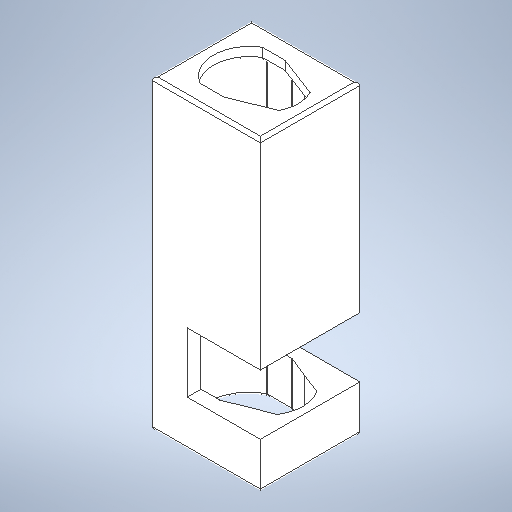
# Autodesk Inventor part: PipetteSleeve
Saved by Autodesk Inventor 2025.1 (Build 291241000, 241)
## iProperties
Created: 2024-10-27
Part Number: PipetteSleeve
Material: Generic
Document SubType Name: Modeling
Designer: 13156
Density: 1 g/cm^3
Appearance: Default
Author: 13156
## iProperties of the stored document PipetteSleeve_3DPrint.ipt
Created: 2024-10-27
Part Number: PipetteSleeve_3DPrint
Material: Generic
Document SubType Name: Modeling
Designer: jerem
Density: 1 g/cm^3
Appearance: Default
Author: jerem
Autodesk Inventor part; units mm, degrees
ref_plane "YZ Plane" through (0, 0, 0) normal (1, 0, 0) x (0, 1, 0)
ref_plane "XZ Plane" through (0, 0, 0) normal (0, 1, 0) x (-1, 0, 0)
ref_plane "XY Plane" through (0, 0, 0) normal (0, 0, 1) x (1, 0, 0)
sketch "Sketch1" plane through (0, 0, 0) normal (0, 1, 0) x (-1, 0, 0)
  arc A0 (11.078, -10.268) -> (11.078, 14.332) centre (5.1039, 2.032) ccw
  line L0 (11.078, -21.6994) -> (11.078, 25.4698)
  line L1 (11.078, 14.332) -> (2.478, 14.332)
  line L2 (11.078, -10.268) -> (2.478, -10.268)
  line L3 (2.478, 14.332) -> (-4.322, 11.532)
  line L4 (2.478, -10.268) -> (-4.322, -7.468)
  line L5 (-4.322, 11.532) -> (-11.422, 8.832)
  line L6 (-4.322, -7.468) -> (-11.422, -4.768)
  arc A1 (-11.422, 8.832) -> (-11.422, -4.768) centre (-0.862, 2.032) ccw
  line L7 (21.1018, 19.039) -> (-15.8982, 19.039)
  line L8 (-15.8982, 19.039) -> (-15.8982, -14.961)
  line L9 (-15.8982, -14.961) -> (21.1018, -14.961)
  line L10 (21.1018, -14.961) -> (21.1018, 19.039)
  point P0 (0, 0)
  point P1 (11.078, 2.032)
  point P2 (18.778, 2.032)
  point P3 (-13.422, 2.032)
  dimension "d0" = 0
  dimension "d1" = 0
  dimension "d2" = 7.7
  dimension "d3" = 8.6
  dimension "d4" = 8.6
  dimension "d5" = 2.8
  dimension "d6" = 2.8
  dimension "d7" = 6.8
  dimension "d8" = 6.8
  dimension "d9" = 24.6
  dimension "d10" = 7.1
  dimension "d11" = 7.1
  dimension "d12" = 2.7
  dimension "d13" = 2.7
  dimension "d14" = 2
  dimension "d56" = 34
  dimension "d57" = 37
  constraints: 22 end point, 6 point on circle, 3 horizontal, 2 centre point, 2 parallel, 1 perpendicular
  measures "d0" vertical distance of point (18.778, 2.032) point (11.078, 2.032)
  measures "d1" distance from line of L0 L1.start
  measures "d2" distance from line of L0 point (18.778, 2.032)
  measures "d3" distance of L1.start L1.end
  measures "d4" distance of L2.start L2.end
  measures "d5" vertical distance of L3.end L1.end
  measures "d6" vertical distance of L4.end L2.end
  measures "d7" horizontal distance of L4.end L2.end
  measures "d8" horizontal distance of L3.end L1.end
  measures "d9" distance of L2.start L1.start
  measures "d10" horizontal distance of L5.end L3.end
  measures "d11" horizontal distance of L6.end L4.end
  measures "d12" vertical distance of L4.end L6.end
  measures "d13" vertical distance of L3.end L5.end
  measures "d14" horizontal distance of L6.end point (-13.422, 2.032)
  measures "d56" distance of L7.end L8.end
  measures "d57" distance of L8.end L9.end
extrude "Extrusion1" add sketch "Sketch1" along normal blind 104.4 contours A0 L0 L7 L10 L9 | L0 L9 L8 L7 L1 L3 L5 A1 L6 L4 L2
sketch "Sketch3" plane through (0, 104.4, 0) normal (0, 1, 0) x (1, 0, 0)
  line L0 (-11.078, -12.682) -> (-2.8044, -12.682)
  line L1 (-2.8044, -12.682) -> (3.6938, -10.0063)
  line L2 (4.322, -11.532) -> (-2.478, -14.332) projected
  line L3 (3.6938, -10.0063) -> (10.43, -7.2326)
  line L4 (10.43, 3.38) -> (-3.3441, 8.618)
  line L5 (-3.3441, 8.618) -> (-11.078, 8.618)
  arc A0 (-11.078, 8.618) -> (-11.078, -12.682) centre (-4.7292, -2.032) ccw
  arc A1 (10.43, -7.2326) -> (10.43, 3.38) centre (0.611, -1.9263) ccw
  line L6 (-2.478, -14.332) -> (-11.078, -14.332) projected
  line L7 (-11.078, 10.268) -> (-2.478, 10.268) projected
  line L8 (4.322, 7.468) -> (11.422, 4.768) projected
  arc A2 (11.422, -8.832) -> (11.422, 4.768) centre (0.862, -2.032) ccw projected
  arc A3 (-11.078, 10.268) -> (-11.078, -14.332) centre (-5.1039, -2.032) ccw projected
  line L9 (-19.5547, -18.0128) -> (14.794, -18.0128)
  line L10 (14.794, -18.0128) -> (14.794, 13.635)
  line L11 (14.794, 13.635) -> (-19.5547, 13.635)
  line L12 (-19.5547, 13.635) -> (-19.5547, -18.0128)
  point P0 (0, 0)
  point P1 (13.422, -2.032)
  point P2 (11.772, -1.9263)
  point P3 (-17.128, -2.032)
  point P4 (-18.778, -2.032)
  dimension "d31" = 1.65
  dimension "d32" = 1.65
  dimension "d33" = 1.65
  dimension "d34" = 180
  dimension "d35" = 1.65
  dimension "d36" = 1.65
  dimension "d37" = 1.65
  dimension "d38" = 0
  constraints: 18 end point, 8 point on circle, 3 horizontal, 3 parallel, 2 centre point, 1 perpendicular, 1 point on line
  measures "d31" distance between parallel lines of L6 L0
  measures "d32" distance between parallel lines of L7 L5
  measures "d33" distance between parallel lines of L1 L2
  measures "d34" angle of L8 L4
  measures "d35" distance from line of L8 L4.start
  measures "d36" horizontal distance of point (13.422, -2.032) point (11.772, -1.926)
  measures "d37" distance of point (-17.128, -2.032) point (-18.778, -2.032)
  measures "d38" horizontal distance of L4.start L3.end
extrude "Extrusion2" add sketch "Sketch3" against normal blind 4
fillet "Fillet2" radius 1 8 edges at (-2.6018, 0, 19.039) (-21.1018, 0, 2.039) (15.8982, 0, 2.039) (-2.6018, 0, -14.961) (-2.6018, 104.4, -14.961) (-21.1018, 104.4, 2.039) (-2.6018, 104.4, 19.039) (15.8982, 104.4, 2.039)
fillet "Fillet3" radius 1 22 edges at (-18.778, 0, 2.032) (-6.778, 0, -10.268) (-6.778, 0, 14.332) (0.922, 0, 12.932) (7.872, 0, 10.182) (13.422, 0, 2.032) (7.872, 0, -6.118) (0.922, 0, -8.868) (-17.128, 100.4, 2.032) (-7.211, 100.4, -8.618) (3.5429, 100.4, -5.999) (11.772, 100.4, 1.9263) (-6.9412, 100.4, 12.682) (3.8128, 100.4, 9.9573) (-11.078, 50.2, 14.332) (-2.478, 50.2, 14.332) (4.322, 50.2, 11.532) (11.422, 50.2, 8.832) (11.422, 50.2, -4.768) (4.322, 50.2, -7.468) (-2.478, 50.2, -10.268) (-11.078, 50.2, -10.268)
sketch "Sketch5" plane through (15.8982, 1, 19.039) normal (1, 0, 0) x (0, 0, -1)
  line L0 (39, 35.2) -> (-4, 35.2)
  line L1 (-4, 35.2) -> (-4, 14.7)
  line L2 (-4, 14.7) -> (39, 14.7)
  line L3 (39, 14.7) -> (39, 35.2)
  line L4 (34, 0) -> (34, 102.4) projected
  line L5 (33, 103.4) -> (1, 103.4) projected
  point P0 (19.039, -1)
  dimension "d58" = 20.5
  dimension "d59" = 5
  dimension "d60" = 43
  dimension "d61" = 88.7
  constraints: 8 end point, 2 parallel, 1 horizontal, 1 perpendicular
  measures "d58" distance of L2.end L0.start
  measures "d59" distance between parallel lines of L4 L3
  measures "d60" distance from line of L1.end L3
  measures "d61" distance between parallel lines of L5 L2
extrude "Extrusion3" cut sketch "Sketch5" against normal blind 25
body "Solid1"
